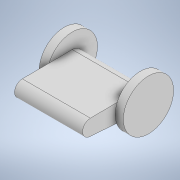
# Autodesk Inventor part: dribbler_sketch001
Saved by Autodesk Inventor 2020 (Build 240168000, 168)
## iProperties
Created: 2024-02-19
Part Number: dribbler_sketch001
Material: Типовые
Document SubType Name: Modeling
Designer: 4s
Density: 1 g/cm^3
Appearance: По умолчанию
Author: 4s
Autodesk Inventor part; units mm, degrees
ref_plane "YZ Plane" through (0, 0, 0) normal (1, 0, 0) x (0, 1, 0)
ref_plane "XZ Plane" through (0, 0, 0) normal (0, 1, 0) x (-1, 0, 0)
ref_plane "XY Plane" through (0, 0, 0) normal (0, 0, 1) x (1, 0, 0)
sketch "Эскиз1" plane through (0, 0, 0) normal (1, 0, 0) x (0, 1, 0)
  circle A0 centre (35.2311, -22.6062) radius 9.3
  circle A1 centre (13.2335, -58.2654) radius 6.1
  circle A2 centre (14.2307, -27.4562) radius 4.85
  circle A3 centre (35.8147, -49.5529) radius 3.55
  line L0 (19.3333, -58.2153) -> (19.0805, -27.4164)
  line L1 (9.3936, -27.1028) -> (7.1497, -57.821)
  point P0 (0, 0)
  dimension "d0" = 18.6
  dimension "d1" = 12.2
  dimension "d2" = 9.7
  dimension "d3" = 7.1
  dimension "d8" = 30.8254
  dimension "d13" = 30.8
  dimension "d14" = 30.8
  constraints: 4 centre point, 4 end point, 4 point on circle, 4 tangent
  measures "d0" diameter of A0
  measures "d1" diameter of A1
  measures "d2" diameter of A2
  measures "d3" diameter of A3
  measures "d8" distance of A1.centre A2.centre
  measures "d13" distance of L0.start L0.end
  measures "d14" distance of L1.start L1.end
extrude "Выдавливание1" add sketch "Эскиз1" along normal blind 42 contours A1 | A1 L1 A2 L0 | A2
sketch "Эскиз2" plane through (42, 0, 0) normal (1, 0, 0) x (0, 0, -1)
  line L0 (27.1028, 9.3936) -> (57.821, 7.1497) construction
  arc A0 (57.821, 7.1497) -> (58.2153, 19.3333) centre (58.2654, 13.2335) ccw construction
  line L1 (58.2153, 19.3333) -> (27.4164, 19.0805) construction
  arc A1 (27.4164, 19.0805) -> (27.1028, 9.3936) centre (27.4562, 14.2307) ccw construction
  circle A2 centre (58.2654, 13.2335) radius 6.1 construction
  circle A3 centre (58.2654, 13.2335) radius 15.5
  point P0 (0, 0)
  dimension "d17" = 31
  constraints: 1 centre point, 1 coincident
  measures "d17" diameter of A3
extrude "Выдавливание2" add sketch "Эскиз2" along normal blind 5
sketch "Эскиз3" plane through (0, 0, 0) normal (-1, 0, 0) x (0, 0, 1)
  line L0 (-27.1028, 9.3936) -> (-57.821, 7.1497) construction
  arc A0 (-27.1028, 9.3936) -> (-27.4164, 19.0805) centre (-27.4562, 14.2307) ccw construction
  line L1 (-58.2153, 19.3333) -> (-27.4164, 19.0805) construction
  arc A1 (-58.2153, 19.3333) -> (-57.821, 7.1497) centre (-58.2654, 13.2335) ccw construction
  circle A2 centre (-58.2654, 13.2335) radius 15.5
  point P0 (0, 0)
  dimension "d20" = 31
  constraints: 1 centre point, 1 coincident
  measures "d20" diameter of A2
extrude "Выдавливание3" add sketch "Эскиз3" along normal blind 5
